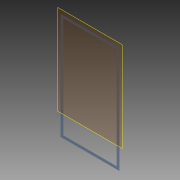
# Autodesk Inventor part: FeederTape
Saved by Autodesk Inventor 2013 (Build 170138000, 138)
## iProperties
Created: 2013-01-04
Part Number: FeederTape
Material: PVC, Unplasticized
Document SubType Name: Modeling
Designer: Phillip
Density: 1 g/cm^3
Author: Phillip
Autodesk Inventor part; units mm, degrees
ref_plane "YZ Plane" through (0, 0, 0) normal (1, 0, 0) x (0, 1, 0)
ref_plane "XZ Plane" through (0, 0, 0) normal (0, 1, 0) x (-1, 0, 0)
ref_plane "XY Plane" through (0, 0, 0) normal (0, 0, 1) x (1, 0, 0)
ref_plane "Work Plane1" through (0, 0, 0) normal (0, 0, 1) x (1, 0, 0)
sketch "Sketch1" plane through (0, 0, 0) normal (0, 0, 1) x (1, 0, 0)
  line L0 (-546.1, 758.825) -> (546.1, 758.825)
  line L1 (546.1, 758.825) -> (546.1, -1222.375)
  line L2 (546.1, -1222.375) -> (-546.1, -1222.375)
  line L3 (-546.1, -1222.375) -> (-546.1, 758.825)
  line L4 (495.3, 708.025) -> (-495.3, 708.025)
  line L5 (-495.3, 708.025) -> (-495.3, -1171.575)
  line L6 (-495.3, -1171.575) -> (495.3, -1171.575)
  line L7 (495.3, -1171.575) -> (495.3, 708.025)
  point P0 (0, 0)
  constraints: 16 end point, 4 parallel, 2 perpendicular, 1 horizontal, 3 other
extrude "Extrusion1" add sketch "Sketch1" along normal blind 0.0254
body "Solid1"
